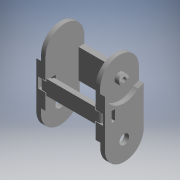
# Autodesk Inventor part: MHPUS306-50-25-Aclip
Saved by Autodesk Inventor 2017.3 (Build 213256000, 256)
## iProperties
Part Number: MHPUS306-50-25-Aclip
Material: Generic
Catalog Web Link: www.cadenas.de
Description: MHPUS_clip-Cable Carriers Flap Open - Close Type
Vendor: MISUMI
Document SubType Name: Modeling
Designer: partserver
Manufacturer: MISUMI
Mass: 30.2003 g
Surface Area: 176.743 cm^2
Volume: 30.2003 cm^3
Density: 1 g/cm^3
Appearance: PSOLRGB-192-192-192
Category: PARTsolutions
Company: MISUMI
Title: MHPUS306-50-25-A
Author: Cadenas PARTsolutions
Comments: Cable Carriers Flap Open - Close Type
PSOL_IDENT_0: {$CADENAS_DATA\23d-libs\misumi\metric\07_slide_rails\mhpus_clip.prj},195 {VTYP=3D},{NB=MHPUS306-50-2
PSOL_IDENT_1: 5-Aclip},{LINA=MHPUS306-50-25-A},{NN=MHPUS_clip},{DATE=30.06.2021 12:53:59},{GEOMDATE=16.03.2015 00:
PSOL_IDENT_2: 00:00},{VERSION=},{LINEID=90},{WBVAR=BR,NOL,AD},{WBNUMERIC=BR,NOL}  {NB=MHPUS306-50-25-Aclip},{LINA=
PSOL_IDENT_3: MHPUS306-50-25-A},{KT=DUMMY},{PN=MHPUS306-50-25-A},{NO=306},{MATB=Nylon 6 + Glass 20 percent},{OTB=-
PSOL_IDENT_4: 10~80},{MATFB=Low Carbon Steel},{STFB=Trivalent Bright Chromate Plating},{BR=50},{BRA=50,100},{NOL=2
PSOL_IDENT_5: 5},{NOLALG=[6-38/1]},{AD=A},{ADALG= 'A', 'Outer circumference', 'B', 'Inner circumference' },{A=24.0
PSOL_IDENT_6: },{B=34},{C=44},{W=60},{P=45},{LL=60},{F=40},{T=24},{J=20},{N=7.0},{P1F=35.6},{P2F=55.6},{P1FX=32},{
PSOL_IDENT_7: P2FX=52},{H=134},{H1=100},{HF=160},{K=257.0},{WT=64.00},{ANGLE=53.48737},{ANGLE2=0.00000},{ANGLE3=90
PSOL_IDENT_8: .00000},{GAMA=27.52031},{GAMA2=0.00000},{GAMA3=nan},{BETA=45.50496},{BETA2=0.00000},{BETA3=0.00000},
PSOL_IDENT_9: {X0=17.00000},{Y0=0.00000},{X1=-28.00000},{Y1=0.00000},{X2=-54.77500},{Y2=36.16766},{X3=-41.63725},{
PSOL_IDENT_10: Y3=79.20717},{X4=0.77167},{Y4=94.25653},{X5=38.10054},{Y5=69.12576},{X6=0.00000},{Y6=0.00000},{X7=0.
PSOL_IDENT_11: 00000},{Y7=100.00000},{X8=45.00000},{Y8=100.00000},{R1=11.5},{R2=8.0},{R3=2.000},{L1=4.000},{L2=19.6
PSOL_IDENT_12: 905},{L3=4.200},{CL1=-26.743683950},{CL2=-53.487367900},{CL3=-53.487367900},{CL4=-42.613450190},{CL5=
PSOL_IDENT_13: -3.668130050},{CL6=0.000000000},{CL7=0},{CL8=0},{CL9=0.000000000},{CL10=0.000000000},{CL11=0.0000000
PSOL_IDENT_14: 00},{CL12=0.000000000},{TILT=0},{MOVE=917},{Z=2}
NB: MHPUS306-50-25-Aclip
NN: MHPUS_clip
NT: Cable Carriers Flap Open - Close Type
NBSYN: $PN.clip
LINA: MHPUS306-50-25-A
CATALOG: Misumi
PN: MHPUS306-50-25-A
NO: 306
MATB: Nylon 6 + Glass 20 percent
OTB: -10~80
MATFB: Low Carbon Steel
STFB: Trivalent Bright Chromate Plating
BR: 50
NOL: 25
AD: Outer circumference
A: 24
B: 34
C: 44
W: 60
P: 45
LL: 60
F: 40
T: 24
J: 20
N: 7
P1F: 35.6
P2F: 55.6
P1FX: 32
P2FX: 52
H: 134
H1: 100
HF: 160
K: 257
WT: 64
R3: 2
SUPPLIER: MISUMI
ARTICLENO: MHPUS306-50-25-Aclip
BOMINFO: MHPUS306-50-25-A
CREATOR: CADENAS GmbH
Autodesk Inventor part; units mm, degrees
sketch "Sketch_1" plane through (0, 0, 0) normal (0, 0, 1) x (1, 0, 0)
  line L0 (-30, 17) -> (-30, -17)
  line L1 (-30, -17) -> (30, -17)
  line L2 (30, -17) -> (30, 17)
  line L3 (30, 17) -> (-30, 17)
  constraints: 8 end point
extrude "Extrusion1" add sketch "Sketch_1" against normal blind 79
sketch "Sketch_3" plane through (0, 0, 0) normal (0, 0, 1) x (1, 0, 0)
  line L0 (-22, 12) -> (-22, -17)
  line L1 (-22, -17) -> (22, -17)
  line L2 (22, -17) -> (22, 12)
  line L3 (22, 12) -> (-22, 12)
  constraints: 8 end point
extrude "Extrusion2" cut sketch "Sketch_3" along normal mid plane 158
sketch "Sketch_6" plane through (0, 0, -31.85) normal (0, 0, 1) x (1, 0, 0)
  line L0 (-13.2, 18.02) -> (-12.289, 14.62)
  line L1 (-12.289, 14.62) -> (12.289, 14.62)
  line L2 (12.289, 14.62) -> (13.2, 18.02)
  line L3 (13.2, 18.02) -> (-13.2, 18.02)
  constraints: 8 end point
extrude "Extrusion3" cut sketch "Sketch_6" against normal blind 18
sketch "Sketch_4" plane through (0, 0, 0) normal (0, 1, 0) x (-1, 0, 0)
  line L0 (60, 60) -> (-60, 60)
  line L1 (-60, 60) -> (-60, -120)
  line L2 (-60, -120) -> (60, -120)
  line L3 (60, -120) -> (60, 60)
  line L4 (30, 0) -> (22, 0)
  line L5 (22, 0) -> (22, -27.2)
  line L6 (22, -27.2) -> (-22, -27.2)
  line L7 (-22, -27.2) -> (-22, 0)
  line L8 (-22, 0) -> (-30, 0)
  line L9 (-30, 0) -> (-30, -79)
  line L10 (-30, -79) -> (-22, -79)
  line L11 (-22, -79) -> (-22, -55.2)
  line L12 (-22, -55.2) -> (22, -55.2)
  line L13 (22, -55.2) -> (22, -79)
  line L14 (22, -79) -> (30, -79)
  line L15 (30, -79) -> (30, 0)
  constraints: 32 end point
extrude "Extrusion4" cut sketch "Sketch_4" along normal mid plane 158
sketch "Sketch_2" plane through (0, 0, 0) normal (1, 0, 0) x (0, 1, 0)
  line L0 (45, 45) -> (-45, 45)
  line L1 (-45, 45) -> (-45, -90)
  line L2 (-45, -90) -> (45, -90)
  line L3 (45, -90) -> (45, 45)
  arc A0 (17, -17) -> (-17, -17) centre (0, -17) ccw
  line L4 (-17, -17) -> (-17, -62)
  arc A1 (-17, -62) -> (17, -62) centre (0, -62) ccw
  line L5 (17, -62) -> (17, -17)
  constraints: 12 end point, 4 point on circle, 2 centre point
extrude "Extrusion5" cut sketch "Sketch_2" along normal mid plane 60
sketch "Sketch_5" plane through (-25.8, 0, 0) normal (1, 0, 0) x (0, 0, -1)
  arc A0 (49.4116, 12.1565) -> (62, -17.5) centre (62, 0) ccw
  line L0 (62, -17.5) -> (62, -56)
  line L1 (62, -56) -> (89.4, -56)
  line L2 (89.4, -56) -> (89.4, 47)
  line L3 (89.4, 47) -> (63.4892, 47)
  line L4 (63.4892, 47) -> (49.4116, 12.1565)
  circle A1 centre (62, 0) radius 4.25
  constraints: 10 end point, 2 centre point, 2 point on circle
extrude "Extrusion6" cut sketch "Sketch_5" against normal blind 15
sketch "Sketch_8" plane through (-25.8, 0, 0) normal (1, 0, 0) x (0, 0, -1)
  circle A0 centre (62, 0) radius 1.8889
  constraints: 1 centre point
extrude "Extrusion7" cut sketch "Sketch_8" against normal blind 15
sketch "Sketch_11" plane through (0, 0, 0) normal (1, 0, 0) x (0, 1, 0)
  circle A0 centre (0, -17) radius 4.25
  constraints: 1 centre point
extrude "Extrusion8" cut sketch "Sketch_11" along normal mid plane 60
sketch "Sketch_24" plane through (-26, 0, 0) normal (1, 0, 0) x (0, 0, -1)
  line L0 (-3.4, -51) -> (17, -51)
  line L1 (17, -51) -> (17, -17.5)
  arc A0 (17, -17.5) -> (29.5884, 12.1565) centre (17, 0) ccw
  line L2 (29.5884, 12.1565) -> (21.5712, 32)
  line L3 (21.5712, 32) -> (-3.4, 32)
  line L4 (-3.4, 32) -> (-3.4, -51)
  constraints: 10 end point, 2 point on circle, 1 centre point
extrude "Extrusion9" cut sketch "Sketch_24" along normal blind 52
sketch "Sketch_7" plane through (25.8, 0, 0) normal (1, 0, 0) x (0, 0, -1)
  arc A0 (49.4116, 12.1565) -> (55.6364, -16.302) centre (62, 0) ccw
  arc A1 (62, -25.6174) -> (55.6364, -16.302) centre (52, -25.6174) ccw
  line L0 (62, -25.6174) -> (62, -56)
  line L1 (62, -56) -> (89.4, -56)
  line L2 (89.4, -56) -> (89.4, 47)
  line L3 (89.4, 47) -> (63.4892, 47)
  line L4 (63.4892, 47) -> (49.4116, 12.1565)
  circle A2 centre (62, 0) radius 4.25
  constraints: 10 end point, 4 point on circle, 3 centre point
extrude "Extrusion10" cut sketch "Sketch_7" along normal blind 15
sketch "Sketch_9" plane through (25.8, 0, 0) normal (1, 0, 0) x (0, 0, -1)
  circle A0 centre (62, 0) radius 1.8889
  constraints: 1 centre point
extrude "Extrusion11" cut sketch "Sketch_9" along normal blind 15
sketch "Sketch_10" plane through (0, 0, -39.5) normal (0, 0, 1) x (1, 0, 0)
  line L0 (-30, -8) -> (-30, -11)
  line L1 (-30, -11) -> (-28.4, -11)
  line L2 (-28.4, -11) -> (-28.4, -17)
  line L3 (-28.4, -17) -> (-22, -17)
  line L4 (-22, -17) -> (-22, -8)
  line L5 (-22, -8) -> (-30, -8)
  circle A0 centre (-24, -12) radius 1.55
  constraints: 12 end point, 1 centre point
extrude "Extrusion12" cut sketch "Sketch_10" along normal mid plane 9
sketch "Sketch_13" plane through (0, 0, -39.5) normal (0, 0, 1) x (1, 0, 0)
  line L0 (22, -8) -> (22, -17)
  line L1 (22, -17) -> (28.4, -17)
  line L2 (28.4, -17) -> (28.4, -11)
  line L3 (28.4, -11) -> (30, -11)
  line L4 (30, -11) -> (30, -8)
  line L5 (30, -8) -> (22, -8)
  circle A0 centre (24, -12) radius 1.55
  constraints: 12 end point, 1 centre point
extrude "Extrusion13" cut sketch "Sketch_13" along normal mid plane 9
sketch "Sketch_14" plane through (0, 0, 0) normal (0, 1, 0) x (-1, 0, 0)
  line L0 (-28.6667, -66.25) -> (-30, -62)
  line L1 (-30, -62) -> (-30, -66.25)
  line L2 (-30, -66.25) -> (-28.6667, -66.25)
  constraints: 6 end point
extrude "Extrusion14" cut sketch "Sketch_14" along normal mid plane 8.5
sketch "Sketch_18" plane through (0, 0, 0) normal (0, 1, 0) x (-1, 0, 0)
  line L0 (30, -62) -> (28.6667, -66.25)
  line L1 (28.6667, -66.25) -> (30, -66.25)
  line L2 (30, -66.25) -> (30, -62)
  constraints: 6 end point
extrude "Extrusion15" cut sketch "Sketch_18" along normal mid plane 8.5
sketch "Sketch_25" plane through (0, 0, -39.5) normal (0, 0, 1) x (1, 0, 0)
  line L0 (-27.4, -9.5) -> (-27.4, -13.4)
  arc A0 (-27.4, -13.4) -> (-23.8, -17) centre (-23.8, -13.4) ccw
  line L1 (-23.8, -17) -> (23.8, -17)
  arc A1 (23.8, -17) -> (27.4, -13.4) centre (23.8, -13.4) ccw
  line L2 (27.4, -13.4) -> (27.4, -9.5)
  line L3 (27.4, -9.5) -> (25.55, -9.5)
  line L4 (25.55, -9.5) -> (25.55, -12)
  arc A2 (22.45, -12) -> (25.55, -12) centre (24, -12) ccw
  line L5 (22.45, -12) -> (-22.45, -12)
  arc A3 (-25.55, -12) -> (-22.45, -12) centre (-24, -12) ccw
  line L6 (-25.55, -12) -> (-25.55, -9.5)
  line L7 (-25.55, -9.5) -> (-27.4, -9.5)
  constraints: 16 end point, 8 point on circle, 4 centre point
extrude "Extrusion16" add sketch "Sketch_25" along normal mid plane 8.1818
sketch "Sketch_27" plane through (0, 0, -39.5) normal (0, 0, 1) x (1, 0, 0)
  arc A0 (-21.2467, -16.6281) -> (-21.1445, -17) centre (-21.1445, -16.8) ccw
  line L0 (-21.1445, -17) -> (21.1445, -17)
  arc A1 (21.1445, -17) -> (21.2467, -16.6281) centre (21.1445, -16.8) ccw
  arc A2 (18.6673, -12.75) -> (21.2467, -16.6281) centre (24, -12) ccw
  line L1 (18.6673, -12.75) -> (-18.6673, -12.75)
  arc A3 (-21.2467, -16.6281) -> (-18.6673, -12.75) centre (-24, -12) ccw
  constraints: 8 point on circle, 4 centre point, 4 end point
extrude "Extrusion17" add sketch "Sketch_27" along normal mid plane 12.8571
ref_plane "clip1_to_dummy_XY" through (0, 0, -17) normal (1, 0, 0) x (0, 0, -1)
ref_plane "clip1_to_dummy_YZ" through (0, 0, -17) normal (0, 0, -1) x (0, 1, 0)
ref_plane "clip1_to_dummy_ZX" through (0, 0, -17) normal (0, 1, 0) x (1, 0, 0)
ref_plane "clip_back_to_clip_front_XY" through (0, 0, -62) normal (1, 0, 0) x (0, 0, -1)
ref_plane "clip_back_to_clip_front_YZ" through (0, 0, -62) normal (0, 0, -1) x (0, 1, 0)
ref_plane "clip_back_to_clip_front_ZX" through (0, 0, -62) normal (0, 1, 0) x (1, 0, 0)
ref_plane "clip_end_to_fitting_free_left_XY" through (-25.8, 0, -917) normal (1, 0, 0) x (0, 0, -1)
ref_plane "clip_end_to_fitting_free_left_YZ" through (-25.8, 0, -917) normal (0, 0, -1) x (0, 1, 0)
ref_plane "clip_end_to_fitting_free_left_ZX" through (-25.8, 0, -917) normal (0, 1, 0) x (1, 0, 0)
ref_plane "clip_end_to_fitting_free_right_XY" through (25.8, 0, -917) normal (1, 0, 0) x (0, 0, -1)
ref_plane "clip_end_to_fitting_free_right_YZ" through (25.8, 0, -917) normal (0, 0, -1) x (0, 1, 0)
ref_plane "clip_end_to_fitting_free_right_ZX" through (25.8, 0, -917) normal (0, 1, 0) x (1, 0, 0)
ref_plane "clip_front_to_clip_back_XY" through (0, 0, -17) normal (1, 0, 0) x (0, 0, -1)
ref_plane "clip_front_to_clip_back_YZ" through (0, 0, -17) normal (0, 0, -1) x (0, 1, 0)
ref_plane "clip_front_to_clip_back_ZX" through (0, 0, -17) normal (0, 1, 0) x (1, 0, 0)
ref_plane "clip_front_to_fitting_fixed_left_XY" through (-26, 0, -17) normal (1, 0, 0) x (0, 0, -1)
ref_plane "clip_front_to_fitting_fixed_left_YZ" through (-26, 0, -17) normal (0, 0, -1) x (0, 1, 0)
ref_plane "clip_front_to_fitting_fixed_left_ZX" through (-26, 0, -17) normal (0, 1, 0) x (1, 0, 0)
ref_plane "clip_front_to_fitting_fixed_right_XY" through (26, 0, -17) normal (1, 0, 0) x (0, 0, -1)
ref_plane "clip_front_to_fitting_fixed_right_YZ" through (26, 0, -17) normal (0, 0, -1) x (0, 1, 0)
ref_plane "clip_front_to_fitting_fixed_right_ZX" through (26, 0, -17) normal (0, 1, 0) x (1, 0, 0)
ref_plane "clip_front_to_fitting_right_XY" through (0, 0, -17) normal (1, 0, 0) x (0, 0, -1)
ref_plane "clip_front_to_fitting_right_YZ" through (0, 0, -17) normal (0, 0, -1) x (0, 1, 0)
ref_plane "clip_front_to_fitting_right_ZX" through (0, 0, -17) normal (0, 1, 0) x (1, 0, 0)
ref_plane "clip_to_flap_XY" through (-24, -12, -39.5) normal (0, 0, 1) x (1, 0, 0)
ref_plane "clip_to_flap_YZ" through (-24, -12, -39.5) normal (1, 0, 0) x (0, 1, 0)
ref_plane "clip_to_flap_ZX" through (-24, -12, -39.5) normal (0, 1, 0) x (0, 0, 1)
ref_plane "to_center_XY" through (0, 44.6514, -39.5) normal (1, 0, 0) x (0, 0, -1)
ref_plane "to_center_YZ" through (0, 44.6514, -39.5) normal (0, 0, -1) x (0, 1, 0)
ref_plane "to_center_ZX" through (0, 44.6514, -39.5) normal (0, 1, 0) x (1, 0, 0)
ref_plane "to_clip1_XY" through (0, 0, -17) normal (0, 0, 1) x (1, 0, 0)
ref_plane "to_clip1_YZ" through (0, 0, -17) normal (1, 0, 0) x (0, 1, 0)
ref_plane "to_clip1_ZX" through (0, 0, -17) normal (0, 1, 0) x (0, 0, 1)
ref_plane "to_clip5_XY" through (0, 0, -917) normal (0, 0, 1) x (1, 0, 0)
ref_plane "to_clip5_YZ" through (0, 0, -917) normal (1, 0, 0) x (0, 1, 0)
ref_plane "to_clip5_ZX" through (0, 0, -917) normal (0, 1, 0) x (0, 0, 1)
body "Solid1"
